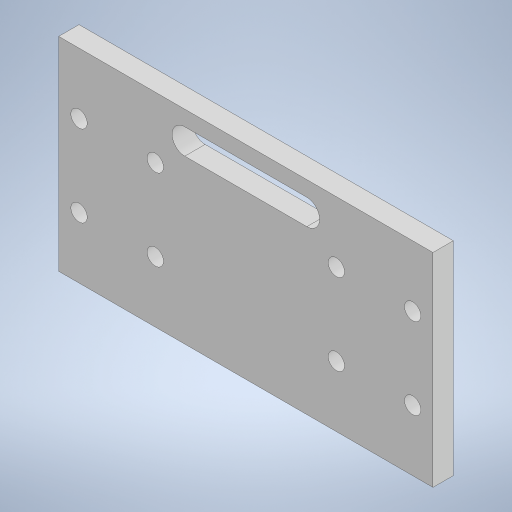
# Autodesk Inventor part: стена_движения_каретки_з
Saved by Autodesk Inventor 2023.1 (Build 271208000, 208)
## iProperties
Created: 2026-02-10
Part Number: стена_движения_каретки_з
Material: Типовые
Document SubType Name: Modeling
Designer: DELL
Density: 1 g/cm^3
Appearance: По умолчанию
Author: DELL
Autodesk Inventor part; units mm, degrees
ref_plane "YZ Plane" through (0, 0, 0) normal (1, 0, 0) x (0, 1, 0)
ref_plane "XZ Plane" through (0, 0, 0) normal (0, 1, 0) x (-1, 0, 0)
ref_plane "XY Plane" through (0, 0, 0) normal (0, 0, 1) x (1, 0, 0)
sketch "Эскиз1" plane through (0, 0, 0) normal (0, 0, 1) x (1, 0, 0)
  line L0 (-36.8, -20) -> (36.8, -20)
  line L1 (36.8, -20) -> (36.8, 20)
  line L2 (36.8, 20) -> (-36.8, 20)
  line L3 (-36.8, 20) -> (-36.8, -20)
  line L4 (-36.8, -20) -> (36.8, 20) construction
  line L5 (36.8, -20) -> (-36.8, 20) construction
  line L6 (-17.8, -8) -> (-32.8, -8) construction
  line L7 (-32.8, -8) -> (-32.8, 8) construction
  line L8 (-32.8, 8) -> (-17.8, 8) construction
  line L9 (-17.8, 8) -> (-17.8, -8) construction
  line L10 (-17.8, -8) -> (-32.8, 8) construction
  line L11 (-32.8, -8) -> (-17.8, 8) construction
  circle A0 centre (-32.8, -8) radius 1.6
  circle A1 centre (-32.8, 8) radius 1.6
  circle A2 centre (-17.8, 8) radius 1.6
  circle A3 centre (-17.8, -8) radius 1.6
  line L12 (0, 0) -> (0, -20) construction
  line L13 (17.8, -8) -> (32.8, -8) construction
  line L14 (32.8, -8) -> (32.8, 8) construction
  line L15 (32.8, 8) -> (17.8, 8) construction
  line L16 (17.8, 8) -> (17.8, -8) construction
  line L17 (17.8, -8) -> (32.8, 8) construction
  line L18 (32.8, -8) -> (17.8, 8) construction
  circle A4 centre (32.8, -8) radius 1.6
  circle A5 centre (32.8, 8) radius 1.6
  circle A6 centre (17.8, 8) radius 1.6
  circle A7 centre (17.8, -8) radius 1.6
  point P0 (-25.3, 0)
  point P1 (25.3, 0)
  dimension "d0" = 73.6
  dimension "d1" = 40
  dimension "d2" = 15
  dimension "d3" = 16
  dimension "d4" = 4
  dimension "d5" = 3.2
  dimension "d6" = 3.2
  dimension "d7" = 3.2
  dimension "d8" = 3.2
  dimension "d9" = 20
  constraints: 38 end point, 9 symmetric about line, 8 centre point, 8 coincident, 5 midpoint, 4 parallel, 2 horizontal, 2 perpendicular, 4 other
  measures "d0" distance of L2.end L1.end
  measures "d1" distance of L2.end L0.start
  measures "d2" distance of L7.end L8.end
  measures "d3" distance of L6.end L7.end
  measures "d4" distance from line of L3 L6.end
  measures "d5" diameter of A0
  measures "d6" diameter of A1
  measures "d7" diameter of A2
  measures "d8" diameter of A3
  measures "d9" distance from line of L0 point (-25.3, 0)
extrude "Выдавливание1" add sketch "Эскиз1" along normal blind 4
sketch "Эскиз2" plane through (0, 0, 4) normal (0, 0, 1) x (1, 0, 0)
  line L0 (-12, 14.5) -> (12, 14.5) construction
  line L1 (-12, 12) -> (12, 12)
  line L2 (12, 17) -> (-12, 17)
  arc A0 (-12, 17) -> (-12, 12) centre (-12, 14.5) ccw
  arc A1 (12, 12) -> (12, 17) centre (12, 14.5) ccw
  line L3 (36.8, 20) -> (-36.8, 20) projected
  point P0 (0, 0)
  point P1 (0, 14.5)
  dimension "d12" = 12
  dimension "d13" = 5
  dimension "d14" = 3
  constraints: 8 end point, 4 point on circle, 4 tangent, 2 centre point, 1 horizontal, 1 midpoint, 1 parallel
  measures "d12" distance of point (0, 14.5) L0.end
  measures "d13" diameter of A1
  measures "d14" distance between parallel lines of L3 L2
extrude "Выдавливание2" cut sketch "Эскиз2" against normal blind 10
